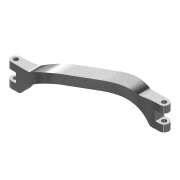
# Autodesk Inventor part: LEG_Dedao
Saved by Autodesk Inventor 2020 (Build 240168000, 168)
## iProperties
Created: 2021-04-01
Part Number: LEG_Dedao
Material: Generic
Document SubType Name: Modeling
Designer: deox
Density: 1 g/cm^3
Appearance: Honed
Author: deox
Autodesk Inventor part; units mm, degrees
ref_plane "YZ Plane" through (0, 0, 0) normal (1, 0, 0) x (0, 1, 0)
ref_plane "XZ Plane" through (0, 0, 0) normal (0, 1, 0) x (-1, 0, 0)
ref_plane "XY Plane" through (0, 0, 0) normal (0, 0, 1) x (1, 0, 0)
sketch "Sketch1" plane through (0, 0, 0) normal (0, 1, 0) x (-1, 0, 0)
  line L0 (17.875, 6.875) -> (-17.875, 6.875)
  line L1 (-17.875, 6.875) -> (-17.875, -6.875)
  line L2 (-17.875, -6.875) -> (17.875, -6.875)
  line L3 (17.875, -6.875) -> (17.875, 6.875)
  line L4 (17.875, 6.875) -> (-17.875, -6.875) construction
  line L5 (-17.875, 6.875) -> (17.875, -6.875) construction
  point P0 (0, 0)
  dimension "d0" = 35.75
  dimension "d1" = 13.75
  constraints: 12 end point, 2 midpoint, 2 parallel, 1 horizontal, 1 perpendicular
  measures "d0" distance of L2.end L1.end
  measures "d1" distance of L1.end L0.end
extrude "Extrusion1" add sketch "Sketch1" along normal blind 8.937
sketch "Sketch2" plane through (0, 8.937, 0) normal (0, 1, 0) x (1, 0, 0)
  line L0 (-18.0794, 7.1815) -> (18.1656, 7.1815) construction
  line L1 (18.1656, 7.1815) -> (18.1656, -7.2125) construction
  line L2 (18.1656, -7.2125) -> (-18.0794, -7.2125) construction
  line L3 (-18.0794, -7.2125) -> (-18.0794, 7.1815) construction
  line L4 (17.875, 6.875) -> (-17.875, 6.875) projected
  line L5 (-17.875, 6.875) -> (-17.875, -6.875) projected
  line L6 (-17.875, -6.875) -> (17.875, -6.875) projected
  line L7 (17.875, -6.875) -> (17.875, 6.875) projected
  line L8 (-17.875, -6.875) -> (17.875, -6.875) projected
  line L9 (-17.875, -6.875) -> (-17.875, -4.125)
  line L10 (-17.875, 6.875) -> (-17.875, -6.875) projected
  line L11 (-17.875, -4.125) -> (-16.5, -4.125)
  line L12 (-16.5, -4.125) -> (-16.5, -5.5)
  circle A0 centre (-16.5, -5.5) radius 1.375
  line L13 (17.875, 6.875) -> (-17.875, 6.875) projected
  line L14 (0, 6.875) -> (0, -6.875)
  line L15 (-11.37, -6.875) -> (-11.37, -3.5364)
  spline S0 degree 3 poles (-16.5, -4.125) (-14.2359, -4.1637) (-13.0998, -3.9579) (-11.37, -3.5364) knots 0 0 0 0 1 1 1 1
  line L16 (0, 0) -> (-1.0312, 1.7862)
  line L17 (0, 0) -> (2.0625, 0) construction
  line L18 (-1.0312, 1.7862) -> (3.8307, 4.5932)
  line L19 (-1.0312, 1.7862) -> (-5.8932, -1.0209)
  line L20 (0, 0) -> (2.032, 1.1732)
  line L21 (0, 0) -> (2.3464, 0) construction
  line L22 (1.0312, -1.7862) -> (5.8932, 1.0209)
  line L23 (1.0312, -1.7862) -> (-3.8307, -4.5932)
  spline S1 degree 4 poles (-11.37, -3.5364) (-10.0636, -3.2214) (-8.1858, -2.397) (-7.6682, -2.1035) (-5.8932, -1.0209) knots 0 0 0 0 0 1 1 1 1 1
  spline S2 degree 4 poles (-11.37, -6.875) (-10.2442, -6.8644) (-9.2661, -6.8622) (-7.4354, -6.4868) (-5.5641, -5.6957) (-4.5883, -5.0303) (-3.8307, -4.5932) knots 0 0 0 0 0 0.420037 0.580947 1 1 1 1 1
  line L24 (-17.875, 0) -> (-12.2961, 0)
  line L25 (-16.5, -6.875) -> (-11.37, -6.875)
  spline S3 degree 4 poles (11.37, 3.5364) (10.056, 3.2168) (8.2023, 2.3998) (7.6448, 2.0947) (5.8932, 1.0209) knots 0 0 0 0 0 1 1 1 1 1
  spline S4 degree 4 poles (11.37, 6.875) (10.2498, 6.8688) (9.2683, 6.8616) (7.4363, 6.4854) (5.5663, 5.6954) (4.5885, 5.0299) (3.8307, 4.5932) knots 0 0 0 0 0 0.419904 0.580884 1 1 1 1 1
  line L26 (11.37, 6.875) -> (11.37, 3.5364)
  line L27 (16.5, 6.875) -> (11.37, 6.875)
  spline S5 degree 3 poles (16.5, 4.125) (14.2269, 4.1544) (13.0995, 3.9572) (11.37, 3.5364) knots 0 0 0 0 1 1 1 1
  line L28 (16.5, 4.125) -> (16.5, 5.5)
  line L29 (17.875, 6.875) -> (17.875, 4.125)
  circle A1 centre (16.5, 5.5) radius 1.375
  circle A2 centre (-16.5, -5.5) radius 0.6874
  circle A3 centre (16.5, 5.5) radius 0.6875
  point P0 (-14.3426, -4.0673)
  point P1 (-12.8976, -3.8725)
  point P2 (-9.9708, -3.0931)
  point P3 (-8.6139, -2.5299)
  point P4 (-7.4703, -1.9519)
  point P5 (-9.737, -6.831)
  point P6 (-8.6072, -6.6839)
  point P7 (-7.4538, -6.389)
  point P8 (-6.2455, -5.9357)
  point P9 (-5.0456, -5.3171)
  point P10 (18.0794, 7.1815)
  point P11 (18.0794, 7.2125)
  point P12 (9.969, 3.0909)
  point P13 (9.7425, 6.8327)
  point P14 (8.6114, 2.5271)
  point P15 (7.4589, 1.9458)
  point P16 (7.4553, 6.3881)
  point P17 (6.2472, 5.9351)
  point P18 (5.0467, 5.3168)
  point P19 (8.6098, 6.6837)
  point P20 (12.894, 3.87)
  point P21 (14.3348, 4.0627)
  point P22 (17.875, 5.5)
  point P23 (16.4657, 4.1254)
  point P24 (-17.875, -5.5)
  point P25 (-16.4548, -4.1257)
  dimension "d27" = 2.75
  dimension "d28" = 1.375
  dimension "d29" = 3.3386
  dimension "d30" = 2.0625
  dimension "d31" = 120
  dimension "d33" = 30
  dimension "d46" = 1.3749
  dimension "d47" = 1.3749
  constraints: 38 end point, 5 symmetric about line, 4 coincident, 4 horizontal, 4 perpendicular, 3 midpoint, 3 point on line, 2 centre point, 2 equal length, 1 parallel, 1 vertical, 40 other
  measures "d27" distance of L5.end L9.end
  measures "d28" distance of L9.end L11.end
  measures "d29" distance of L15.start L15.end
  measures "d30" distance of L16.start L16.end
  measures "d31" angle of L17 L16
  measures "d33" angle of L21 L20
  measures "d46" diameter of A2
  measures "d47" diameter of A3
extrude "Extrusion2" cut sketch "Sketch2" against normal blind 8.937 contours L7 A1 L4 | A3 | A1 L7 L6 L14 L23 L22 S3 S5 | S4 L18 L14 L4 | L14 L18 L19 S1 S0 L11 L5 L4 | L6 S2 L23 L14 | L11 A0 L5 | A2 | L6 L5 A0
sketch "Sketch3" plane through (-16.5, 0, 6.875) normal (0, 0, 1) x (1, 0, 0)
  line L0 (-1.375, 0) -> (-1.375, 8.937) projected
  line L1 (-1.375, 0) -> (0.0452, 0) projected
  line L2 (0, 0) -> (5.13, 0) projected
  line L3 (12.6693, 0) -> (5.13, 0) projected
  line L4 (22.3932, 0) -> (12.6693, 0) projected
  line L5 (27.87, 0) -> (22.3932, 0) projected
  line L6 (32.9657, 0) -> (27.87, 0) projected
  line L7 (32.9657, 0) -> (34.375, 0) projected
  line L8 (34.375, 0) -> (34.375, 8.937) projected
  line L9 (34.375, 8.937) -> (32.9657, 8.937) projected
  line L10 (27.87, 8.937) -> (32.9657, 8.937) projected
  line L11 (22.3932, 8.937) -> (27.87, 8.937) projected
  line L12 (12.6693, 8.937) -> (22.3932, 8.937) projected
  line L13 (5.13, 8.937) -> (12.6693, 8.937) projected
  line L14 (0, 8.937) -> (5.13, 8.937) projected
  line L15 (0.0452, 8.937) -> (-1.375, 8.937) projected
  line L16 (-1.5183, 9.706) -> (35.0687, 9.706) construction
  line L17 (35.0687, 9.706) -> (35.0687, -0.8431) construction
  line L18 (35.0687, -0.8431) -> (-1.5183, -0.8431) construction
  line L19 (-1.5183, -0.8431) -> (-1.5183, 9.706) construction
  line L20 (-1.375, 0) -> (-1.375, 2.035)
  line L21 (-1.375, 2.035) -> (1.152, 2.035)
  line L22 (1.402, 2.285) -> (1.402, 4.585)
  line L23 (1.152, 4.835) -> (-1.375, 4.835)
  line L24 (-1.375, 4.835) -> (-1.375, 6.87)
  line L25 (-1.375, 6.87) -> (5.3179, 6.87)
  line L26 (-1.375, 0) -> (34.375, 0)
  line L27 (33, 0) -> (27.87, 0) projected
  line L28 (16.5, 0) -> (16.5, 8.937)
  line L29 (20.3307, 8.937) -> (10.6068, 8.937) projected
  arc A0 (2.0563, 0) -> (3.0513, 0.5945) centre (2.0563, 1.13) ccw
  line L30 (16.5, 8.937) -> (16.5, 6.187)
  line L31 (16.5, 6.187) -> (12.6693, 6.187)
  line L32 (12.6693, 8.937) -> (12.6693, 0) projected
  arc A1 (12.6693, 6.187) -> (3.0513, 0.5945) centre (12.6693, -4.8798) ccw
  arc A2 (12.6693, 8.937) -> (5.3179, 6.87) centre (12.6693, -5.1693) ccw
  arc A3 (1.402, 4.585) -> (1.152, 4.835) centre (1.152, 4.585) ccw
  arc A4 (1.152, 2.035) -> (1.402, 2.285) centre (1.152, 2.285) ccw
  line L33 (34.375, 0) -> (34.375, 8.937)
  line L34 (34.375, 0) -> (32.9548, 0)
  line L35 (33, 0) -> (27.87, 0)
  line L36 (20.3307, 0) -> (27.87, 0)
  line L37 (27.87, 8.937) -> (20.3307, 8.937)
  line L38 (33, 8.937) -> (27.87, 8.937)
  line L39 (32.9548, 8.937) -> (34.375, 8.937)
  line L40 (34.375, 0) -> (34.375, 2.035)
  line L41 (34.375, 2.035) -> (31.848, 2.035)
  line L42 (31.598, 2.285) -> (31.598, 4.585)
  line L43 (31.848, 4.835) -> (34.375, 4.835)
  line L44 (34.375, 4.835) -> (34.375, 6.87)
  line L45 (34.375, 6.87) -> (27.6821, 6.87)
  arc A5 (29.9487, 0.5945) -> (30.9437, 0) centre (30.9437, 1.13) ccw
  line L46 (20.3307, 8.937) -> (20.3307, 0)
  arc A6 (29.9487, 0.5945) -> (20.3307, 6.187) centre (20.3307, -4.8798) ccw
  arc A7 (27.6821, 6.87) -> (20.3307, 8.937) centre (20.3307, -5.1693) ccw
  arc A8 (31.848, 4.835) -> (31.598, 4.585) centre (31.848, 4.585) ccw
  arc A9 (31.598, 2.285) -> (31.848, 2.035) centre (31.848, 2.285) ccw
  line L47 (16.5, 6.187) -> (20.3307, 6.187)
  line L48 (20.3307, 8.937) -> (20.3307, 0) projected
  line L49 (16.5, 8.937) -> (20.3307, 8.937)
  point P0 (1.402, 2.035)
  point P1 (1.402, 4.835)
  point P2 (34.5183, 9.706)
  point P3 (31.598, 2.035)
  point P4 (31.598, 4.835)
  point P5 (2.0563, 0)
  point P6 (30.9437, 0)
  dimension "d67" = 2.035
  dimension "d68" = 2.777
  dimension "d69" = 2.8
  dimension "d70" = 2.035
  dimension "d71" = 2.75
  dimension "d73" = 0.25
  constraints: 52 end point, 22 symmetric about line, 20 point on circle, 19 point on line, 10 centre point, 8 tangent, 6 perpendicular, 2 collinear, 1 equal radius, 1 horizontal, 7 other
  measures "d67" distance of L0.start L20.end
  measures "d68" distance of L20.end point (1.402, 2.035)
  measures "d69" distance of point (1.402, 2.035) point (1.402, 4.835)
  measures "d70" distance of L23.end L24.end
  measures "d71" distance of L28.end L30.end
  measures "d73" radius of A3
extrude "Extrusion3" cut sketch "Sketch3" against normal through all contours L0 L23 A3 L22 A4 L21 | L0 L15 L14 L13 A2 L25 | A0 A1 L32 L3 L2 | L32 L31 L28 L4 | L28 L47 L46 L4 | L12 L11 L10 L9 L8 L45 A7 | L46 A6 A5 L6 L5 L4 | L8 L41 A9 L42 A8 L43
fillet "Fillet1" radius 2 2 edges at (-11.1821, 6.87, 5.1808) (11.1821, 6.87, -5.181)
sketch "Sketch4" plane through (-3.8307, 6.187, -0.1699) normal (0, -1, 0) x (1, 0, 0)
  line L0 (3.8307, 0.1699) -> (0.8537, 1.8887)
  line L1 (3.8307, 0.1699) -> (8.6432, 0.1699) construction
  line L2 (3.8307, 0.1699) -> (4.7111, 1.6948)
  line L3 (-0.3371, 2.5762) -> (0.3504, 3.767)
  line L4 (0.3504, 3.767) -> (4.5182, 1.3607)
  line L5 (-1.0246, 1.3854) -> (3.1432, -1.0209)
  arc A0 (0.3504, 3.767) -> (-1.0246, 1.3854) centre (-0.3371, 2.5762) ccw
  line L6 (3.8307, 0.1699) -> (6.8076, -1.5488)
  line L7 (7.9984, -2.2363) -> (8.6859, -1.0455)
  line L8 (8.6859, -1.0455) -> (4.5182, 1.3607)
  line L9 (7.3109, -3.4271) -> (3.1432, -1.0209)
  arc A1 (7.3109, -3.4271) -> (8.6859, -1.0455) centre (7.9984, -2.2363) ccw
  dimension "d79" = 4.8125
  dimension "d80" = 150
  dimension "d81" = 1.375
  constraints: 20 end point, 7 symmetric about line, 6 point on circle, 2 centre point, 2 coincident, 1 horizontal, 1 perpendicular, 1 point on line, 1 other
  measures "d79" distance of L0.start L3.start
  measures "d80" angle of L1 L0
  measures "d81" distance of L3.end L3.start
extrude "Extrusion4" cut sketch "Sketch4" along normal blind 0.75 and the other way blind 0.7327
body "Solid1"
